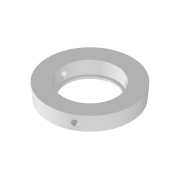
# Autodesk Inventor part: 50_Filteradapter_Fluorescence_CCVTV_Berrybase_100mm
Saved by Autodesk Inventor 2022 (Build 260153000, 153)
## iProperties
Created: 2023-04-26
Part Number: 50_Filteradapter_Fluorescence_CCVTV_Berrybase_100mm
Material: Generisch
Document SubType Name: Modeling
Designer: diederichbenedict
Density: 1 g/cm^3
Appearance: Vorgabe
Author: diederichbenedict
Autodesk Inventor part; units mm, degrees
ref_plane "YZ Plane" through (0, 0, 0) normal (1, 0, 0) x (0, 1, 0)
ref_plane "XZ Plane" through (0, 0, 0) normal (0, 1, 0) x (-1, 0, 0)
ref_plane "XY Plane" through (0, 0, 0) normal (0, 0, 1) x (1, 0, 0)
sketch "Skizze1" plane through (0, 0, 0) normal (0, 1, 0) x (-1, 0, 0)
  circle A0 centre (0, 0) radius 19.5
  line L0 (-8, 0) -> (8, 0) construction
  circle A1 centre (0, 0) radius 11.5
  dimension "d0" = 39
  dimension "d1" = 8
  dimension "d8" = 23
  constraints: 4 end point, 2 centre point, 2 coincident, 1 horizontal, 1 midpoint
  measures "d0" diameter of A0
  measures "d1" distance of A0.centre L0.end
  measures "d8" diameter of A1
extrude "Extrusion1" add sketch "Skizze1" along normal blind 7 draft 5
sketch "Skizze2" plane through (0, 7, 0) normal (0, 1, 0) x (1, 0, 0)
  circle A0 centre (0, 0) radius 20.1124 projected
  circle A1 centre (0, 0) radius 12.8
  dimension "d5" = 25.6
  constraints: 1 centre point, 1 coincident
  measures "d5" diameter of A1
extrude "Extrusion2" cut sketch "Skizze2" against normal blind 6 contours A1
sketch "Skizze3" plane through (0, 0, 0) normal (1, 0, 0) x (0, 1, 0)
  line L0 (7, 20.1124) -> (7, -20.1124) projected
  line L1 (0, -19.5) -> (0, 19.5) projected
  circle A0 centre (3.3414, 0) radius 1.45
  point P0 (0, 0)
  dimension "d9" = 2.9
  constraints: 1 centre point
  measures "d9" diameter of A0
extrude "Extrusion3" cut sketch "Skizze3" against normal through all
pattern_circular "Runde Anordnung1" count 3 over 360 about axis through (0, 7, 0) along (0, -1, 0) of "Extrusion3"
